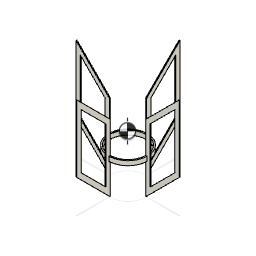
Rocket_Airframe_Fins_LL v3 (Autodesk Fusion 360 archive; units mm, degrees)
design "SIngle_Fin_2mm_Thickness_Square_Cuts"
Autodesk Fusion 360 part; units mm, degrees
sketch "Sketch1" plane through (0, 0, 0) normal (0, 1, 0) x (1, 0, 0)
  line L0 (1, 41.0878) -> (1, 117.3)
  line L1 (-1, 41.0878) -> (-1, 117.3)
  line L2 (-1, 117.3) -> (1, 117.3)
  arc A0 (1, 41.0878) -> (-1, 41.0878) centre (0, 0) ccw
  constraint coincident A0.centre origin
  constraint perpendicular L0 L2
extrude "Extrude1" add sketch "Sketch1" along normal blind 152.4 makes body 1
sketch "Sketch2" plane through (1, 0, 0) normal (1, 0, 0) x (0, 0, -1)
  line L0 (41.0878, 0) -> (117.3, 0)
  line L1 (117.3, 0) -> (117.3, 152.4)
  line L2 (117.3, 152.4) -> (41.0878, 152.4)
  line L3 (41.0878, 152.4) -> (41.0878, 0)
  line L4 (41.0878, 0) -> (117.3, 76.2122)
  line L5 (41.0878, 0) -> (148.8681, 0) construction
  line L6 (117.3, 0) -> (41.0878, 0)
  line L7 (117.3, 0) -> (117.3, 3.3314)
  line L8 (117.3, 0) -> (117.3, 76.2122)
  dimension "d7" = 45
  constraint horizontal L5
  constraint coincident L0.start L3.end
  constraint coincident L1 L4.end
  constraint coincident L0.end L1.start
  constraint coincident L1 L7.end
  measures "d7" angle of L4 L5
extrude "Extrude2" cut sketch "Sketch2" against normal blind 10 contours L0 L1 L4 L6 L7 L8 bodies 1
sketch "Sketch3" plane through (1, 0, 0) normal (1, 0, 0) x (0, 0, -1)
  line L0 (41.0878, 0) -> (117.3, 76.2122)
  line L1 (117.3, 76.2122) -> (117.3, 152.4)
  line L2 (117.3, 152.4) -> (41.0878, 152.4)
  line L3 (41.0878, 152.4) -> (41.0878, 0)
  line L4 (41.0878, 152.4) -> (117.3, 228.6122)
  line L5 (41.0878, 152.4) -> (148.8681, 152.4) construction
  line L6 (117.3, 228.6122) -> (117.3, 152.4)
  line L7 (41.0878, 152.4) -> (117.3, 152.4)
  dimension "d10" = 45
  constraint horizontal L5
  constraint coincident L2.end L3.start
  constraint coincident L1.end L2.start
  constraint perpendicular L2 L6
  measures "d10" angle of L4 L5
extrude "Extrude3" add sketch "Sketch3" against normal blind 2 contours L2 L4 L6 L7 bodies 1
sketch "Sketch5" plane through (1, 0, 0) normal (1, 0, 0) x (0, 0, -1)
  line L0 (41.0878, 0) -> (117.3, 76.2122)
  line L1 (117.3, 76.2122) -> (117.3, 228.6122)
  line L2 (117.3, 228.6122) -> (41.0878, 152.4)
  line L3 (41.0878, 152.4) -> (41.0878, 0)
  line L4 (51.0878, 148.2579) -> (107.3, 204.47)
  line L5 (107.3, 80.3543) -> (107.3, 204.47)
  line L6 (107.3, 80.3543) -> (51.0878, 24.1421)
  line L7 (51.0878, 148.2579) -> (51.0878, 24.1421)
extrude "Extrude5" cut sketch "Sketch5" against normal blind 10 contours L4 L5 L6 L7 bodies 1
sketch "Sketch7" plane through (1, 0, 0) normal (1, 0, 0) x (0, 0, -1)
  line L0 (51.0878, 148.2579) -> (107.3, 204.47)
  line L1 (107.3, 204.47) -> (107.3, 80.3543)
  line L2 (107.3, 80.3543) -> (51.0878, 24.1421)
  line L3 (51.0878, 24.1421) -> (51.0878, 148.2579)
  line L4 (41.0878, 0) -> (117.3, 76.2122)
  line L5 (117.3, 76.2122) -> (117.3, 228.6122)
  line L6 (117.3, 228.6122) -> (41.0878, 152.4)
  line L7 (41.0878, 152.4) -> (41.0878, 0)
  line L8 (41.0878, 81.2) -> (41.0878, 76.2)
  line L9 (41.0878, 71.2) -> (44.0878, 71.2)
  line L10 (44.0878, 71.2) -> (44.0878, 81.2)
  line L11 (44.0878, 81.2) -> (41.0878, 81.2)
  line L12 (38.0878, 71.2) -> (44.0878, 81.2) construction
  line L13 (44.0878, 71.2) -> (38.0878, 81.2) construction
  line L14 (41.0878, 71.2) -> (41.0878, 76.2)
  point P0 (41.0878, 76.2)
  dimension "d49" = 6
  dimension "d50" = 10
  constraint midpoint L7 P0
  constraint horizontal L9
  constraint perpendicular L9 L10
  constraint parallel L9 L11
  constraint coincident L12 P0
  constraint coincident L13 P0
  constraint coincident P0 L8.end
  constraint coincident L7 L9.start
  measures "d49" distance of L10.end L13.end
  measures "d50" distance of L9.end L10.end
extrude "Extrude6" cut sketch "Sketch7" against normal blind 3 contours L7 L8 L9 L10 L11 L14 bodies 1
sketch "Sketch8" plane through (0, 71.2, 0) normal (0, 1, 0) x (-1, 0, 0)
  arc A0 (-1, -41.0878) -> (1, -41.0878) centre (0, 0) ccw
  line L0 (-1, -41.0878) -> (-1, -44.0878)
  line L1 (-1, -44.0878) -> (1, -44.0878)
  line L2 (1, -44.0878) -> (1, -41.0878)
  circle A1 centre (0, 0) radius 41.1
  circle A2 centre (0, 0) radius 44.1
  dimension "d53" = 82.2
  dimension "d54" = 3
  constraint concentric A0 A1
  measures "d53" diameter of A1
extrude "Extrude7" add sketch "Sketch8" along normal blind 10 contours A0 L0 L1 L2 A1 | L0 L2 A1 A2 | L1 A2 bodies 1
pattern_circular "C-Pattern1" count 4 over 360 about axis through (0, 1.75, 0) along (0, 1, 0) of "Extrude1", "Extrude2", "Extrude3", "Extrude5", "Extrude6" makes body 2 at (-113.9667, 169.7648, -1) makes body 3 at (-1, 169.7648, 113.9667) makes body 4 at (113.9667, 169.7648, 1)
